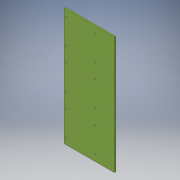
# Autodesk Inventor part: GBX_002.1-bottom-plate
Saved by Autodesk Inventor 2019 (Build 230136000, 136)
## iProperties
Created: 2019-08-15
Part Number: GBX_002.1-bottom-plate
Material: Generic
Document SubType Name: Modeling
Designer: Rene
Density: 1 g/cm^3
Appearance: Olive Green
Author: Rene
Autodesk Inventor part; units mm, degrees
ref_plane "YZ Plane" through (0, 0, 0) normal (1, 0, 0) x (0, 1, 0)
ref_plane "XZ Plane" through (0, 0, 0) normal (0, 1, 0) x (-1, 0, 0)
ref_plane "XY Plane" through (0, 0, 0) normal (0, 0, 1) x (1, 0, 0)
sketch "Sketch1" plane through (0, 0, 0) normal (0, 0, 1) x (1, 0, 0)
  line L0 (150, -350) -> (-150, -350)
  line L1 (-150, -350) -> (-150, 350)
  line L2 (-150, 350) -> (150, 350)
  line L3 (150, 350) -> (150, -350)
  line L4 (150, -350) -> (-150, 350) construction
  line L5 (-150, -350) -> (150, 350) construction
  point P0 (0, 0)
  dimension "d0" = 700
  dimension "d1" = 300
  constraints: 12 end point, 2 midpoint, 2 parallel, 1 horizontal, 1 perpendicular
  measures "d0" distance of L0.end L1.end
  measures "d1" distance of L1.end L2.end
extrude "Extrusion1" add sketch "Sketch1" along normal blind 9
sketch "Sketch2" plane through (0, 0, 9) normal (0, 0, 1) x (1, 0, 0)
  line L0 (-135, -162.5) -> (35, -162.5) construction
  line L1 (35, -162.5) -> (35, -312.5) construction
  line L2 (35, -312.5) -> (-135, -312.5) construction
  line L3 (-135, -312.5) -> (-135, -162.5) construction
  point P0 (0, 0)
  point P1 (-150, -350)
  dimension "d4" = 170
  dimension "d5" = 150
  dimension "d16" = 37.5
  dimension "d17" = 15
  constraints: 8 end point, 3 coincident, 2 parallel, 1 horizontal, 1 perpendicular
  measures "d4" distance of L0.start L0.end
  measures "d5" distance of L0.end L1.end
  measures "d16" vertical distance of point (-135, -312.5) point (-150, -350)
  measures "d17" horizontal distance of point (-135, -312.5) point (-150, -350)
hole "Hole1" at (35, -162.5, 9) at (35, -312.5, 9) at (-135, -162.5, 9) at (-135, -312.5, 9) direction (0, 0, -1) diameter 5 end through all
mirror "Mirror1" about plane through (0, 0, 0) normal (0, 1, 0) of "Hole1"
sketch "Sketch4" plane through (0, 0, 9) normal (0, 0, 1) x (1, 0, 0)
  line L0 (-135, 75) -> (35, 75) construction
  line L1 (35, 75) -> (35, -75) construction
  line L2 (35, -75) -> (-135, -75) construction
  line L3 (-135, -75) -> (-135, 75) construction
  circle A0 centre (35, 162.5) radius 2.5 construction
  circle A1 centre (-135, 162.5) radius 2.5 construction
  circle A2 centre (35, 312.5) radius 2.5 construction
  circle A3 centre (35, -162.5) radius 2.5 construction
  point P0 (0, 0)
  dimension "d18" = 150
  dimension "d19" = 170
  dimension "d20" = 170
  dimension "d21" = 150
  dimension "d22" = 87.5
  dimension "d23" = 87.5
  dimension "d24" = 0
  constraints: 8 end point, 4 coincident, 2 parallel, 1 horizontal, 1 perpendicular
  measures "d18" distance of L0.end L1.end
  measures "d19" distance of L0.start L0.end
  measures "d20" distance of A0.centre A1.centre
  measures "d21" distance of A0.centre A2.centre
  measures "d22" distance of L0.end A0.centre
  measures "d23" distance of A3.centre L1.end
  measures "d24" horizontal distance of A0.centre L0.end
hole "Hole2" at (35, 75, 9) at (35, -75, 9) at (-135, -75, 9) at (-135, 75, 9) direction (0, 0, -1) diameter 5 end through all
equation "\"d18\" = d21"
equation "\"d19\" = d20"
body "Solid1"
